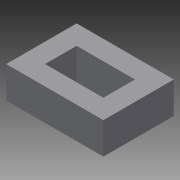
# Autodesk Inventor part: grommet
Saved by Autodesk Inventor 2014 SP1 (Build 180222100, 222)
## iProperties
Created: 2014-06-18
Part Number: grommet
Material: Generic
Document SubType Name: Modeling
Designer: Nick
Density: 1 g/cm^3
Appearance: Default
Author: Nick
Autodesk Inventor part; units mm, degrees
ref_plane "YZ Plane" through (0, 0, 0) normal (1, 0, 0) x (0, 1, 0)
ref_plane "XZ Plane" through (0, 0, 0) normal (0, 1, 0) x (-1, 0, 0)
ref_plane "XY Plane" through (0, 0, 0) normal (0, 0, 1) x (1, 0, 0)
sketch "Sketch1" plane through (0, 0, 0) normal (0, 0, 1) x (1, 0, 0)
  line L0 (0, 0) -> (10, 0)
  line L1 (10, 0) -> (10, 7.25)
  line L2 (10, 7.25) -> (0, 7.25)
  line L3 (0, 7.25) -> (0, 0)
  line L4 (2, 5.25) -> (8, 5.25)
  line L5 (8, 5.25) -> (8, 2)
  line L6 (8, 2) -> (2, 2)
  line L7 (2, 2) -> (2, 5.25)
  dimension "d0" = 10
  dimension "d1" = 7.25
  dimension "d7" = 2
  constraints: 16 end point, 4 parallel, 2 perpendicular, 1 horizontal, 3 other
  measures "d0" distance of L2.end L1.end
  measures "d1" distance of L1.end L0.end
  measures "d7" distance between parallel lines of L2 L4
extrude "Extrusion1" add sketch "Sketch1" along normal blind 3.25
body "Solid1"
